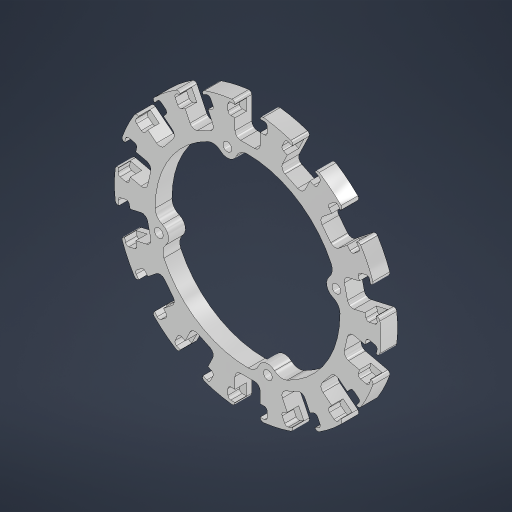
# Autodesk Inventor part: OmniFrame_D
Saved by Autodesk Inventor 2024.2 (Build 282272000, 272)
## iProperties
Created: 2024-02-19
Part Number: OmniFrame_D
Material: 一般
Document SubType Name: Modeling
Designer: Hanaoka
Density: 1 g/cm^3
Appearance: 既定
Author: Hanaoka
Autodesk Inventor part; units mm, degrees
ref_plane "YZ Plane" through (0, 0, 0) normal (1, 0, 0) x (0, 1, 0)
ref_plane "XZ Plane" through (0, 0, 0) normal (0, 1, 0) x (-1, 0, 0)
ref_plane "XY Plane" through (0, 0, 0) normal (0, 0, 1) x (1, 0, 0)
sketch "スケッチ1" plane through (0, 0, 0) normal (0, 0, 1) x (1, 0, 0)
  circle A0 centre (0, 0) radius 25 construction
  line L0 (-2.25, 24.8985) -> (-2.25, 19)
  line L1 (-1.25, 18) -> (1.25, 18)
  line L2 (2.25, 19) -> (2.25, 24.8985)
  line L3 (0, 25) -> (0, 18) construction
  line L4 (-2.25, 23.025) -> (-3, 23.025)
  line L5 (-3.5, 22.525) -> (-3.5, 21.475)
  line L6 (-3, 20.975) -> (-2.25, 20.975)
  line L7 (2.25, 23.025) -> (3, 23.025)
  line L8 (3.5, 22.525) -> (3.5, 21.475)
  line L9 (3, 20.975) -> (2.25, 20.975)
  arc A1 (-3, 23.025) -> (-3.5, 22.525) centre (-3, 22.525) ccw
  arc A2 (-3.5, 21.475) -> (-3, 20.975) centre (-3, 21.475) ccw
  arc A3 (3.5, 22.525) -> (3, 23.025) centre (3, 22.525) ccw
  arc A4 (3, 20.975) -> (3.5, 21.475) centre (3, 21.475) ccw
  arc A5 (-2.25, 19) -> (-1.25, 18) centre (-1.25, 19) ccw
  arc A6 (1.25, 18) -> (2.25, 19) centre (1.25, 19) ccw
  arc A7 (-10.271, 16.1422) -> (-8.9361, 15.6751) centre (-9.37, 16.5761) ccw
  arc A8 (-6.6837, 16.7598) -> (-6.2166, 18.0946) centre (-7.1176, 17.6608) ccw
  line L10 (-8.9361, 15.6751) -> (-6.6837, 16.7598)
  line L11 (-6.3978, 20.1995) -> (-7.0735, 19.8741)
  arc A9 (-6.3978, 20.1995) -> (-6.1643, 20.8669) centre (-6.6147, 20.65) ccw
  line L12 (-6.6198, 21.8129) -> (-6.1643, 20.8669)
  arc A10 (-6.6198, 21.8129) -> (-7.2873, 22.0465) centre (-7.0703, 21.596) ccw
  line L13 (-7.963, 21.721) -> (-7.2873, 22.0465)
  line L14 (-11.8036, 17.5962) -> (-11.1279, 17.9216)
  line L15 (-6.2166, 18.0946) -> (-8.7759, 23.4091)
  line L16 (-10.8471, 22.5242) -> (-7.8099, 16.2174) construction
  line L17 (-12.8303, 21.4566) -> (-10.271, 16.1422)
  arc A11 (-12.471, 17.8297) -> (-11.8036, 17.5962) centre (-12.0206, 18.0467) ccw
  line L18 (-12.0174, 19.7686) -> (-12.6931, 19.4432)
  line L19 (-12.9266, 18.7757) -> (-12.471, 17.8297)
  arc A12 (-12.6931, 19.4432) -> (-12.9266, 18.7757) centre (-12.4761, 18.9927) ccw
  arc A13 (-16.2577, 10.0872) -> (-14.8523, 10.2455) centre (-15.6342, 10.869) ccw
  arc A14 (-13.2936, 12.2001) -> (-13.4519, 13.6054) centre (-14.0754, 12.8236) ccw
  line L20 (-14.8523, 10.2455) -> (-13.2936, 12.2001)
  line L21 (-14.5284, 15.4232) -> (-14.9961, 14.8368)
  arc A15 (-14.5284, 15.4232) -> (-14.6076, 16.1259) centre (-14.9194, 15.7349) ccw
  line L22 (-15.4285, 16.7805) -> (-14.6076, 16.1259)
  arc A16 (-15.4285, 16.7805) -> (-16.1312, 16.7013) centre (-15.7403, 16.3896) ccw
  line L23 (-16.5988, 16.115) -> (-16.1312, 16.7013)
  line L24 (-18.2694, 10.7322) -> (-17.8018, 11.3186)
  line L25 (-13.4519, 13.6054) -> (-18.0636, 17.2831)
  line L26 (-19.5458, 15.5872) -> (-14.073, 11.2228) construction
  line L27 (-20.8693, 13.7649) -> (-16.2577, 10.0872)
  arc A17 (-18.972, 10.653) -> (-18.2694, 10.7322) centre (-18.6603, 11.0439) ccw
  line L28 (-19.4045, 12.5967) -> (-19.8721, 12.0104)
  line L29 (-19.793, 11.3077) -> (-18.972, 10.653)
  arc A18 (-19.8721, 12.0104) -> (-19.793, 11.3077) centre (-19.4812, 11.6986) ccw
  arc A19 (-19.0243, 2.0343) -> (-17.8269, 2.7867) centre (-18.8018, 3.0092) ccw
  arc A20 (-17.2706, 5.224) -> (-18.023, 6.4215) centre (-18.2455, 5.4466) ccw
  line L30 (-17.8269, 2.7867) -> (-17.2706, 5.224)
  line L31 (-19.7816, 7.5922) -> (-19.9484, 6.861)
  arc A21 (-19.7816, 7.5922) -> (-20.1578, 8.1909) centre (-20.269, 7.7034) ccw
  line L32 (-21.1814, 8.4245) -> (-20.1578, 8.1909)
  arc A22 (-21.1814, 8.4245) -> (-21.7802, 8.0483) centre (-21.2927, 7.9371) ccw
  line L33 (-21.947, 7.3171) -> (-21.7802, 8.0483)
  line L34 (-21.1167, 1.7426) -> (-20.9498, 2.4738)
  line L35 (-18.023, 6.4215) -> (-23.7736, 7.734)
  line L36 (-24.3732, 5.563) -> (-17.5487, 4.0054) construction
  line L37 (-24.775, 3.3469) -> (-19.0243, 2.0343)
  arc A23 (-21.7154, 1.3664) -> (-21.1167, 1.7426) centre (-21.6041, 1.8539) ccw
  line L38 (-22.9484, 2.93) -> (-23.1153, 2.1988)
  line L39 (-22.7391, 1.6) -> (-21.7154, 1.3664)
  arc A24 (-23.1153, 2.1988) -> (-22.7391, 1.6) centre (-22.6278, 2.0875) ccw
  arc A25 (-18.023, -6.4215) -> (-17.2706, -5.224) centre (-18.2455, -5.4466) ccw
  arc A26 (-17.8269, -2.7867) -> (-19.0243, -2.0343) centre (-18.8018, -3.0092) ccw
  line L40 (-17.2706, -5.224) -> (-17.8269, -2.7867)
  line L41 (-21.1167, -1.7426) -> (-20.9498, -2.4738)
  arc A27 (-21.1167, -1.7426) -> (-21.7154, -1.3664) centre (-21.6041, -1.8539) ccw
  line L42 (-22.7391, -1.6) -> (-21.7154, -1.3664)
  arc A28 (-22.7391, -1.6) -> (-23.1153, -2.1988) centre (-22.6278, -2.0875) ccw
  line L43 (-22.9484, -2.93) -> (-23.1153, -2.1988)
  line L44 (-19.7816, -7.5922) -> (-19.9484, -6.861)
  line L45 (-19.0243, -2.0343) -> (-24.775, -3.3469)
  line L46 (-24.3732, -5.563) -> (-17.5487, -4.0054) construction
  line L47 (-23.7736, -7.734) -> (-18.023, -6.4215)
  arc A29 (-20.1578, -8.1909) -> (-19.7816, -7.5922) centre (-20.269, -7.7034) ccw
  line L48 (-21.947, -7.3171) -> (-21.7802, -8.0483)
  line L49 (-21.1814, -8.4245) -> (-20.1578, -8.1909)
  arc A30 (-21.7802, -8.0483) -> (-21.1814, -8.4245) centre (-21.2927, -7.9371) ccw
  arc A31 (-13.4519, -13.6054) -> (-13.2936, -12.2001) centre (-14.0754, -12.8236) ccw
  arc A32 (-14.8523, -10.2455) -> (-16.2577, -10.0872) centre (-15.6342, -10.869) ccw
  line L50 (-13.2936, -12.2001) -> (-14.8523, -10.2455)
  line L51 (-18.2694, -10.7322) -> (-17.8018, -11.3186)
  arc A33 (-18.2694, -10.7322) -> (-18.972, -10.653) centre (-18.6603, -11.0439) ccw
  line L52 (-19.793, -11.3077) -> (-18.972, -10.653)
  arc A34 (-19.793, -11.3077) -> (-19.8721, -12.0104) centre (-19.4812, -11.6986) ccw
  line L53 (-19.4045, -12.5967) -> (-19.8721, -12.0104)
  line L54 (-14.5284, -15.4232) -> (-14.9961, -14.8368)
  line L55 (-16.2577, -10.0872) -> (-20.8693, -13.7649)
  line L56 (-19.5458, -15.5872) -> (-14.073, -11.2228) construction
  line L57 (-18.0636, -17.2831) -> (-13.4519, -13.6054)
  arc A35 (-14.6076, -16.1259) -> (-14.5284, -15.4232) centre (-14.9194, -15.7349) ccw
  line L58 (-16.5988, -16.115) -> (-16.1312, -16.7013)
  line L59 (-15.4285, -16.7805) -> (-14.6076, -16.1259)
  arc A36 (-16.1312, -16.7013) -> (-15.4285, -16.7805) centre (-15.7403, -16.3896) ccw
  arc A37 (-6.2166, -18.0946) -> (-6.6837, -16.7598) centre (-7.1176, -17.6608) ccw
  arc A38 (-8.9361, -15.6751) -> (-10.271, -16.1422) centre (-9.37, -16.5761) ccw
  line L60 (-6.6837, -16.7598) -> (-8.9361, -15.6751)
  line L61 (-11.8036, -17.5962) -> (-11.1279, -17.9216)
  arc A39 (-11.8036, -17.5962) -> (-12.471, -17.8297) centre (-12.0206, -18.0467) ccw
  line L62 (-12.9266, -18.7757) -> (-12.471, -17.8297)
  arc A40 (-12.9266, -18.7757) -> (-12.6931, -19.4432) centre (-12.4761, -18.9927) ccw
  line L63 (-12.0174, -19.7686) -> (-12.6931, -19.4432)
  line L64 (-6.3978, -20.1995) -> (-7.0735, -19.8741)
  line L65 (-10.271, -16.1422) -> (-12.8303, -21.4566)
  line L66 (-10.8471, -22.5242) -> (-7.8099, -16.2174) construction
  line L67 (-8.7759, -23.4091) -> (-6.2166, -18.0946)
  arc A41 (-6.1643, -20.8669) -> (-6.3978, -20.1995) centre (-6.6147, -20.65) ccw
  line L68 (-7.963, -21.721) -> (-7.2873, -22.0465)
  line L69 (-6.6198, -21.8129) -> (-6.1643, -20.8669)
  arc A42 (-7.2873, -22.0465) -> (-6.6198, -21.8129) centre (-7.0703, -21.596) ccw
  arc A43 (2.25, -19) -> (1.25, -18) centre (1.25, -19) ccw
  arc A44 (-1.25, -18) -> (-2.25, -19) centre (-1.25, -19) ccw
  line L70 (1.25, -18) -> (-1.25, -18)
  line L71 (-3, -20.975) -> (-2.25, -20.975)
  arc A45 (-3, -20.975) -> (-3.5, -21.475) centre (-3, -21.475) ccw
  line L72 (-3.5, -22.525) -> (-3.5, -21.475)
  arc A46 (-3.5, -22.525) -> (-3, -23.025) centre (-3, -22.525) ccw
  line L73 (-2.25, -23.025) -> (-3, -23.025)
  line L74 (3, -20.975) -> (2.25, -20.975)
  line L75 (-2.25, -19) -> (-2.25, -24.8985)
  line L76 (0, -25) -> (0, -18) construction
  line L77 (2.25, -24.8985) -> (2.25, -19)
  arc A47 (3.5, -21.475) -> (3, -20.975) centre (3, -21.475) ccw
  line L78 (2.25, -23.025) -> (3, -23.025)
  line L79 (3.5, -22.525) -> (3.5, -21.475)
  arc A48 (3, -23.025) -> (3.5, -22.525) centre (3, -22.525) ccw
  arc A49 (10.271, -16.1422) -> (8.9361, -15.6751) centre (9.37, -16.5761) ccw
  arc A50 (6.6837, -16.7598) -> (6.2166, -18.0946) centre (7.1176, -17.6608) ccw
  line L80 (8.9361, -15.6751) -> (6.6837, -16.7598)
  line L81 (6.3978, -20.1995) -> (7.0735, -19.8741)
  arc A51 (6.3978, -20.1995) -> (6.1643, -20.8669) centre (6.6147, -20.65) ccw
  line L82 (6.6198, -21.8129) -> (6.1643, -20.8669)
  arc A52 (6.6198, -21.8129) -> (7.2873, -22.0465) centre (7.0703, -21.596) ccw
  line L83 (7.963, -21.721) -> (7.2873, -22.0465)
  line L84 (11.8036, -17.5962) -> (11.1279, -17.9216)
  line L85 (6.2166, -18.0946) -> (8.7759, -23.4091)
  line L86 (10.8471, -22.5242) -> (7.8099, -16.2174) construction
  line L87 (12.8303, -21.4566) -> (10.271, -16.1422)
  arc A53 (12.471, -17.8297) -> (11.8036, -17.5962) centre (12.0206, -18.0467) ccw
  line L88 (12.0174, -19.7686) -> (12.6931, -19.4432)
  line L89 (12.9266, -18.7757) -> (12.471, -17.8297)
  arc A54 (12.6931, -19.4432) -> (12.9266, -18.7757) centre (12.4761, -18.9927) ccw
  arc A55 (16.2577, -10.0872) -> (14.8523, -10.2455) centre (15.6342, -10.869) ccw
  arc A56 (13.2936, -12.2001) -> (13.4519, -13.6054) centre (14.0754, -12.8236) ccw
  line L90 (14.8523, -10.2455) -> (13.2936, -12.2001)
  line L91 (14.5284, -15.4232) -> (14.9961, -14.8368)
  arc A57 (14.5284, -15.4232) -> (14.6076, -16.1259) centre (14.9194, -15.7349) ccw
  line L92 (15.4285, -16.7805) -> (14.6076, -16.1259)
  arc A58 (15.4285, -16.7805) -> (16.1312, -16.7013) centre (15.7403, -16.3896) ccw
  line L93 (16.5988, -16.115) -> (16.1312, -16.7013)
  line L94 (18.2694, -10.7322) -> (17.8018, -11.3186)
  line L95 (13.4519, -13.6054) -> (18.0636, -17.2831)
  line L96 (19.5458, -15.5872) -> (14.073, -11.2228) construction
  line L97 (20.8693, -13.7649) -> (16.2577, -10.0872)
  arc A59 (18.972, -10.653) -> (18.2694, -10.7322) centre (18.6603, -11.0439) ccw
  line L98 (19.4045, -12.5967) -> (19.8721, -12.0104)
  line L99 (19.793, -11.3077) -> (18.972, -10.653)
  arc A60 (19.8721, -12.0104) -> (19.793, -11.3077) centre (19.4812, -11.6986) ccw
  arc A61 (19.0243, -2.0343) -> (17.8269, -2.7867) centre (18.8018, -3.0092) ccw
  arc A62 (17.2706, -5.224) -> (18.023, -6.4215) centre (18.2455, -5.4466) ccw
  line L100 (17.8269, -2.7867) -> (17.2706, -5.224)
  line L101 (19.7816, -7.5922) -> (19.9484, -6.861)
  arc A63 (19.7816, -7.5922) -> (20.1578, -8.1909) centre (20.269, -7.7034) ccw
  line L102 (21.1814, -8.4245) -> (20.1578, -8.1909)
  arc A64 (21.1814, -8.4245) -> (21.7802, -8.0483) centre (21.2927, -7.9371) ccw
  line L103 (21.947, -7.3171) -> (21.7802, -8.0483)
  line L104 (21.1167, -1.7426) -> (20.9498, -2.4738)
  line L105 (18.023, -6.4215) -> (23.7736, -7.734)
  line L106 (24.3732, -5.563) -> (17.5487, -4.0054) construction
  line L107 (24.775, -3.3469) -> (19.0243, -2.0343)
  arc A65 (21.7154, -1.3664) -> (21.1167, -1.7426) centre (21.6041, -1.8539) ccw
  line L108 (22.9484, -2.93) -> (23.1153, -2.1988)
  line L109 (22.7391, -1.6) -> (21.7154, -1.3664)
  arc A66 (23.1153, -2.1988) -> (22.7391, -1.6) centre (22.6278, -2.0875) ccw
  arc A67 (18.023, 6.4215) -> (17.2706, 5.224) centre (18.2455, 5.4466) ccw
  arc A68 (17.8269, 2.7867) -> (19.0243, 2.0343) centre (18.8018, 3.0092) ccw
  line L110 (17.2706, 5.224) -> (17.8269, 2.7867)
  line L111 (21.1167, 1.7426) -> (20.9498, 2.4738)
  arc A69 (21.1167, 1.7426) -> (21.7154, 1.3664) centre (21.6041, 1.8539) ccw
  line L112 (22.7391, 1.6) -> (21.7154, 1.3664)
  arc A70 (22.7391, 1.6) -> (23.1153, 2.1988) centre (22.6278, 2.0875) ccw
  line L113 (22.9484, 2.93) -> (23.1153, 2.1988)
  line L114 (19.7816, 7.5922) -> (19.9484, 6.861)
  line L115 (19.0243, 2.0343) -> (24.775, 3.3469)
  line L116 (24.3732, 5.563) -> (17.5487, 4.0054) construction
  line L117 (23.7736, 7.734) -> (18.023, 6.4215)
  arc A71 (20.1578, 8.1909) -> (19.7816, 7.5922) centre (20.269, 7.7034) ccw
  line L118 (21.947, 7.3171) -> (21.7802, 8.0483)
  line L119 (21.1814, 8.4245) -> (20.1578, 8.1909)
  arc A72 (21.7802, 8.0483) -> (21.1814, 8.4245) centre (21.2927, 7.9371) ccw
  arc A73 (13.4519, 13.6054) -> (13.2936, 12.2001) centre (14.0754, 12.8236) ccw
  arc A74 (14.8523, 10.2455) -> (16.2577, 10.0872) centre (15.6342, 10.869) ccw
  line L120 (13.2936, 12.2001) -> (14.8523, 10.2455)
  line L121 (18.2694, 10.7322) -> (17.8018, 11.3186)
  arc A75 (18.2694, 10.7322) -> (18.972, 10.653) centre (18.6603, 11.0439) ccw
  line L122 (19.793, 11.3077) -> (18.972, 10.653)
  arc A76 (19.793, 11.3077) -> (19.8721, 12.0104) centre (19.4812, 11.6986) ccw
  line L123 (19.4045, 12.5967) -> (19.8721, 12.0104)
  line L124 (14.5284, 15.4232) -> (14.9961, 14.8368)
  line L125 (16.2577, 10.0872) -> (20.8693, 13.7649)
  line L126 (19.5458, 15.5872) -> (14.073, 11.2228) construction
  line L127 (18.0636, 17.2831) -> (13.4519, 13.6054)
  arc A77 (14.6076, 16.1259) -> (14.5284, 15.4232) centre (14.9194, 15.7349) ccw
  line L128 (16.5988, 16.115) -> (16.1312, 16.7013)
  line L129 (15.4285, 16.7805) -> (14.6076, 16.1259)
  arc A78 (16.1312, 16.7013) -> (15.4285, 16.7805) centre (15.7403, 16.3896) ccw
  arc A79 (6.2166, 18.0946) -> (6.6837, 16.7598) centre (7.1176, 17.6608) ccw
  arc A80 (8.9361, 15.6751) -> (10.271, 16.1422) centre (9.37, 16.5761) ccw
  line L130 (6.6837, 16.7598) -> (8.9361, 15.6751)
  line L131 (11.8036, 17.5962) -> (11.1279, 17.9216)
  arc A81 (11.8036, 17.5962) -> (12.471, 17.8297) centre (12.0206, 18.0467) ccw
  line L132 (12.9266, 18.7757) -> (12.471, 17.8297)
  arc A82 (12.9266, 18.7757) -> (12.6931, 19.4432) centre (12.4761, 18.9927) ccw
  line L133 (12.0174, 19.7686) -> (12.6931, 19.4432)
  line L134 (6.3978, 20.1995) -> (7.0735, 19.8741)
  line L135 (10.271, 16.1422) -> (12.8303, 21.4566)
  line L136 (10.8471, 22.5242) -> (7.8099, 16.2174) construction
  line L137 (8.7759, 23.4091) -> (6.2166, 18.0946)
  arc A83 (6.1643, 20.8669) -> (6.3978, 20.1995) centre (6.6147, 20.65) ccw
  line L138 (7.963, 21.721) -> (7.2873, 22.0465)
  line L139 (6.6198, 21.8129) -> (6.1643, 20.8669)
  arc A84 (7.2873, 22.0465) -> (6.6198, 21.8129) centre (7.0703, 21.596) ccw
  circle A85 centre (0, 0) radius 23.75
  circle A86 centre (0, 0) radius 16.5
  line L140 (-3.616, 15.8426) -> (0, 0) construction
  line L141 (0, 0) -> (0, 16.5) construction
  circle A87 centre (0, 0) radius 14.5
  circle A88 centre (-3.616, 15.8426) radius 0.8
  circle A89 centre (-3.616, 15.8426) radius 1.75
  circle A90 centre (0, 0) radius 18 construction
  line L142 (0, 0) -> (-16.5, 0) construction
  circle A91 centre (-15.8426, -3.616) radius 1.75
  circle A92 centre (-15.8426, -3.616) radius 0.8
  line L143 (0, 0) -> (0, -16.5) construction
  circle A93 centre (3.616, -15.8426) radius 1.75
  circle A94 centre (3.616, -15.8426) radius 0.8
  line L144 (0, 0) -> (16.5, 0) construction
  circle A95 centre (15.8426, 3.616) radius 1.75
  circle A96 centre (15.8426, 3.616) radius 0.8
  point P0 (-2.25, 18)
  point P1 (2.25, 18)
  point P2 (3.5, 23.025)
  point P3 (3.5, 20.975)
  point P4 (-3.5, 22)
  point P5 (-9.8371, 15.2412)
  point P6 (-5.7827, 17.1937)
  point P7 (-5.9473, 20.4164)
  point P8 (-6.8368, 22.2634)
  point P9 (-12.6988, 18.3027)
  point P10 (-15.4758, 9.4637)
  point P11 (-12.6701, 12.9819)
  point P12 (-14.2167, 15.8141)
  point P13 (-15.8195, 17.0923)
  point P14 (-19.3825, 10.9804)
  point P15 (-18.0494, 1.8118)
  point P16 (-17.048, 6.199)
  point P17 (-19.6703, 8.0796)
  point P18 (-21.6689, 8.5358)
  point P19 (-22.2272, 1.4832)
  point P20 (-17.048, -6.199)
  point P21 (-18.0494, -1.8118)
  point P22 (-21.2279, -1.2551)
  point P23 (-23.2265, -1.7113)
  point P24 (-20.6696, -8.3077)
  point P25 (-12.6701, -12.9819)
  point P26 (-15.4758, -9.4637)
  point P27 (-18.5811, -10.3413)
  point P28 (-20.1839, -11.6194)
  point P29 (-15.0181, -16.4532)
  point P30 (-5.7827, -17.1937)
  point P31 (-9.8371, -15.2412)
  point P32 (-12.2541, -17.3792)
  point P33 (-13.1436, -19.2262)
  point P34 (-6.3921, -21.3399)
  point P35 (2.25, -18)
  point P36 (-2.25, -18)
  point P37 (-3.5, -20.975)
  point P38 (-3.5, -23.025)
  point P39 (3.5, -22)
  point P40 (9.8371, -15.2412)
  point P41 (5.7827, -17.1937)
  point P42 (5.9473, -20.4164)
  point P43 (6.8368, -22.2634)
  point P44 (12.6988, -18.3027)
  point P45 (15.4758, -9.4637)
  point P46 (12.6701, -12.9819)
  point P47 (14.2167, -15.8141)
  point P48 (15.8195, -17.0923)
  point P49 (19.3825, -10.9804)
  point P50 (18.0494, -1.8118)
  point P51 (17.048, -6.199)
  point P52 (19.6703, -8.0796)
  point P53 (21.6689, -8.5358)
  point P54 (22.2272, -1.4832)
  point P55 (17.048, 6.199)
  point P56 (18.0494, 1.8118)
  point P57 (21.2279, 1.2551)
  point P58 (23.2265, 1.7113)
  point P59 (20.6696, 8.3077)
  point P60 (12.6701, 12.9819)
  point P61 (15.4758, 9.4637)
  point P62 (18.5811, 10.3413)
  point P63 (20.1839, 11.6194)
  point P64 (15.0181, 16.4532)
  point P65 (5.7827, 17.1937)
  point P66 (9.8371, 15.2412)
  point P67 (12.2541, 17.3792)
  point P68 (13.1436, 19.2262)
  point P69 (6.3921, 21.3399)
  point P70 (-4.7759, 22.5432)
  point P71 (-10.7571, 21.178)
  point P72 (-14.8115, 19.2255)
  point P73 (-19.6081, 15.4004)
  point P74 (-22.4138, 11.8822)
  point P75 (-25.0757, 6.3547)
  point P76 (-26.077, 1.9675)
  point P77 (-26.077, -4.1675)
  point P78 (-25.0757, -8.5547)
  point P79 (-22.4138, -14.0822)
  point P80 (-19.6081, -17.6004)
  point P81 (-14.8115, -21.4255)
  point P82 (-10.7571, -23.378)
  point P83 (-4.7759, -24.7432)
  point P84 (-0.2759, -24.7432)
  point P85 (5.7053, -23.378)
  point P86 (9.7596, -21.4255)
  point P87 (14.5562, -17.6004)
  point P88 (17.3619, -14.0822)
  point P89 (20.0238, -8.5547)
  point P90 (21.0251, -4.1675)
  point P91 (21.0251, 1.9675)
  point P92 (20.0238, 6.3547)
  point P93 (17.3619, 11.8822)
  point P94 (14.5562, 15.4004)
  point P95 (9.7596, 19.2255)
  point P96 (5.7053, 21.178)
  point P97 (-0.2759, 22.5432)
  point P98 (-0.7759, 15.15)
  point P99 (14.3838, 0.65)
  point P100 (13.7241, 0.65)
  point P101 (13.7241, -2.85)
  point P102 (14.3838, -2.85)
  point P103 (-0.7759, -18.0097)
  point P104 (-0.7759, -17.35)
  point P105 (-4.2759, -17.35)
  point P106 (-4.2759, -18.0097)
  point P107 (-19.4356, -2.85)
  point P108 (-18.7759, -2.85)
  point P109 (-18.7759, 0.65)
  point P110 (-19.4356, 0.65)
  point P111 (-4.2759, 15.15)
  point P112 (-0.7759, 13.294)
  point P113 (11.8681, 0.65)
  point P114 (11.8681, -2.85)
  point P115 (-0.7759, -15.494)
  point P116 (-4.2759, -15.494)
  point P117 (-16.9199, -2.85)
  point P118 (-16.9199, 0.65)
  point P119 (-4.2759, 13.294)
  point P120 (-2.5259, -15.6)
  point P121 (11.9741, -1.1)
  point P122 (-17.0259, -1.1)
  point P123 (-2.5259, 13.4)
  point P124 (22.5497, 7.4547)
  point P125 (19.8878, 12.9822)
  point P126 (17.0821, 16.5004)
  point P127 (12.2856, 20.3255)
  point P128 (8.2312, 22.278)
  point P129 (2.25, 23.6432)
  point P130 (-2.25, 23.6432)
  point P131 (-8.2312, 22.278)
  point P132 (-12.2856, 20.3255)
  point P133 (-17.0821, 16.5004)
  point P134 (-19.8878, 12.9822)
  point P135 (-22.5497, 7.4547)
  point P136 (-23.5511, 3.0675)
  point P137 (-23.5511, -3.0675)
  point P138 (-22.5497, -7.4547)
  point P139 (-19.8878, -12.9822)
  point P140 (-17.0821, -16.5004)
  point P141 (-12.2856, -20.3255)
  point P142 (-8.2312, -22.278)
  point P143 (-2.25, -23.6432)
  point P144 (2.25, -23.6432)
  point P145 (8.2312, -22.278)
  point P146 (12.2856, -20.3255)
  point P147 (17.0821, -16.5004)
  point P148 (19.8878, -12.9822)
  point P149 (22.5497, -7.4547)
  point P150 (23.5511, -3.0675)
  point P151 (23.5511, 3.0675)
  point P152 (-15.8986, -4.414)
  point P153 (-16.2393, -2.9213)
  point P154 (16.2393, 2.9213)
  point P155 (15.8986, 4.414)
  point P156 (2.9213, -16.2393)
  point P157 (4.414, -15.8986)
  point P158 (-1.9519, 16.3841)
  point P159 (15.6085, 5.3502)
  point P160 (14.1365, 3.2266)
  point P161 (3.2266, -14.1365)
  point P162 (1.9519, -16.3841)
  point P163 (-15.6085, -5.3502)
  point P164 (-16.3841, -1.9519)
  point P165 (-5.3502, 15.6085)
  point P166 (16.3841, 1.9519)
  point P167 (5.3502, -15.6085)
  dimension "d15" = 47.5
  dimension "d16" = 33
  dimension "d6" = 50
  dimension "d7" = 4.5
  dimension "d8" = 0.5
  dimension "d9" = 2.05
  dimension "d11" = 1
  dimension "d12" = 7
  dimension "d13" = 3
  dimension "d14" = 360
  dimension "d28" = 12.857
  dimension "d35" = 1.6
  dimension "d36" = 3.5
  dimension "d45" = 360
  dimension "d49" = 6
  constraints: 290 end point, 224 point on line, 171 point on circle, 94 centre point, 13 tangent, 12 coincident, 5 perpendicular, 4 equal radius, 2 equal length, 2 midpoint, 2 vertical, 1 horizontal, 1 parallel, 697 other
  measures "d6" diameter of A0
  measures "d7" distance of point (-2.25, 18) point (2.25, 18)
  measures "d8" radius of A1
  measures "d9" distance between parallel lines of L6 L4
  measures "d11" radius of A5
  measures "d12" distance of L3.start L3.end
  measures "d13" vertical distance of point (-3.5, 22) L3.start
  measures "d28" angle of L141 L140
  measures "d35" diameter of A88
  measures "d36" diameter of A89
  measures "d49" distance of A3.centre A1.centre
extrude "押し出し1" add sketch "スケッチ1" along normal blind 2.05 contours L4 A1 L5 A2 L6 L0 A5 L1 A6 L2 L9 A4 L8 A3 L7 A85 L137 L138 A84 L139 A83 L134 A79 L130 A80 L135 L131 A81 L132 A82 L133 L127 L128 A78 L129 A77 L124 A73 L120 A74 L125 L121 A75 L122 A76 L123 L117 L118 A72 L119 A71 L114 A67 L110 A95 A86 A89 A91 L40 A26 L45 L41 A27 L42 A28 L43 L37 L38 A24 L39 A23 L34 A19 L30 A20 L35 L31 A21 L32 A22 L33 L27 L28 A18 L29 A17 L24 A13 L20 A14 L25 L21 A15 L22 A16 L23 L17 L18 A12 L19 A11 L14 A7 L10 A8 L15 L11 A9 L12 A10 L13 | A85 L107 L108 A66 L109 A65 L104 A61 L100 A62 L105 L101 A63 L102 A64 L103 L97 L98 A60 L99 A59 L94 A55 L90 A56 L95 L91 A57 L92 A58 L93 L87 L88 A54 L89 A53 L84 A49 L80 A50 L85 L81 A51 L82 A52 L83 L77 L78 A48 L79 A47 L74 A43 L70 A44 L75 L71 A45 L72 A46 L73 L67 L68 A42 L69 A41 L64 A37 L60 A38 L65 L61 A39 L62 A40 L63 L57 L58 A36 L59 A35 L54 A31 L50 A32 L55 L51 A33 L52 A34 L53 L47 L48 A30 L49 A29 L44 A25 L40 A91 A86 A93 A95 L110 A68 L115 L111 A69 L112 A70 L113 | A95 A86 A96 | A86 A96 A95 | A91 A86 A92 | A89 A86 A88 | A86 A88 A89 | A91 A86 A92 | A93 A86 A94 | A86 A94 A93
extrude "押し出し2" add sketch "スケッチ1" against normal blind 0.95 contours L4 A1 L5 A2 L6 L0 A5 L1 A6 L2 L9 A4 L8 A3 L7 A85 L137 L138 A84 L139 A83 L134 A79 L130 A80 L135 L131 A81 L132 A82 L133 L127 L128 A78 L129 A77 L124 A73 L120 A74 L125 L121 A75 L122 A76 L123 L117 L118 A72 L119 A71 L114 A67 L110 A95 A86 A89 A91 L40 A26 L45 L41 A27 L42 A28 L43 L37 L38 A24 L39 A23 L34 A19 L30 A20 L35 L31 A21 L32 A22 L33 L27 L28 A18 L29 A17 L24 A13 L20 A14 L25 L21 A15 L22 A16 L23 L17 L18 A12 L19 A11 L14 A7 L10 A8 L15 L11 A9 L12 A10 L13 | L0 L6 A2 L5 A1 L4 | L7 A3 L8 A4 L9 L2 | L13 A10 L12 A9 L11 L15 | L137 L134 A83 L139 A84 L138 | L17 L14 A11 L19 A12 L18 | L133 A82 L132 A81 L131 L135 | L23 A16 L22 A15 L21 L25 | L127 L124 A77 L129 A78 L128 | L27 L24 A17 L29 A18 L28 | L123 A76 L122 A75 L121 L125 | L33 A22 L32 A21 L31 L35 | L117 L114 A71 L119 A72 L118 | A85 L107 L108 A66 L109 A65 L104 A61 L100 A62 L105 L101 A63 L102 A64 L103 L97 L98 A60 L99 A59 L94 A55 L90 A56 L95 L91 A57 L92 A58 L93 L87 L88 A54 L89 A53 L84 A49 L80 A50 L85 L81 A51 L82 A52 L83 L77 L78 A48 L79 A47 L74 A43 L70 A44 L75 L71 A45 L72 A46 L73 L67 L68 A42 L69 A41 L64 A37 L60 A38 L65 L61 A39 L62 A40 L63 L57 L58 A36 L59 A35 L54 A31 L50 A32 L55 L51 A33 L52 A34 L53 L47 L48 A30 L49 A29 L44 A25 L40 A91 A86 A93 A95 L110 A68 L115 L111 A69 L112 A70 L113 | L37 L34 A23 L39 A24 L38 | L113 A70 L112 A69 L111 L115 | L43 A28 L42 A27 L41 L45 | L47 L44 A29 L49 A30 L48 | L107 L104 A65 L109 A66 L108 | L53 A34 L52 A33 L51 L55 | A95 A86 A96 | L103 A64 L102 A63 L101 L105 | L57 L54 A35 L59 A36 L58 | A86 A96 A95 | L97 L94 A59 L99 A60 L98 | A91 A86 A92 | L63 A40 L62 A39 L61 L65 | A89 A86 A88 | A86 A88 A89 | L93 A58 L92 A57 L91 L95 | A91 A86 A92 | L67 L64 A41 L69 A42 L68 | L87 L84 A53 L89 A54 L88 | A93 A86 A94 | A86 A94 A93 | L73 A46 L72 A45 L71 L75 | L83 A52 L82 A51 L81 L85 | L77 L74 A47 L79 A48 L78
fillet "フィレット1" radius 0.5 28 edges at (-2.25, 23.6432, 0.55) (-8.2312, 22.278, 0.55) (-12.2856, 20.3255, 0.55) (-17.0821, 16.5004, 0.55) (-19.8878, 12.9822, 0.55) (-22.5497, 7.4547, 0.55) (-23.5511, 3.0675, 0.55) (-23.5511, -3.0675, 0.55) (-22.5497, -7.4547, 0.55) (-19.8878, -12.9822, 0.55) (-17.0821, -16.5004, 0.55) (-12.2856, -20.3255, 0.55) (-8.2312, -22.278, 0.55) (-2.25, -23.6432, 0.55) (2.25, -23.6432, 0.55) (8.2312, -22.278, 0.55) (12.2856, -20.3255, 0.55) (17.0821, -16.5004, 0.55) (19.8878, -12.9822, 0.55) (23.5511, -3.0675, 0.55) (22.5497, -7.4547, 0.55) (23.5511, 3.0675, 0.55) (19.8878, 12.9822, 0.55) (17.0821, 16.5004, 0.55) (12.2856, 20.3255, 0.55) (8.2312, 22.278, 0.55) (2.25, 23.6432, 0.55) (22.5497, 7.4547, 0.55)
fillet "フィレット2" radius 2 8 edges at (-15.6085, -5.3502, 0.55) (-16.3841, -1.9519, 0.55) (1.9519, -16.3841, 0.55) (5.3502, -15.6085, 0.55) (16.3841, 1.9519, 0.55) (15.6085, 5.3502, 0.55) (-5.3502, 15.6085, 0.55) (-1.9519, 16.3841, 0.55)
